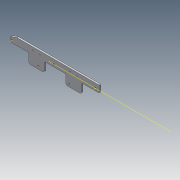
# Autodesk Inventor part: VP CAP SIDE COMP GUIDE
Saved by Autodesk Inventor 2020.3 (Build 243373000, 373)
## iProperties
RuleStatus: InUse
AfterDocSave0: file://Part Number Cleaner
Created: 2018-10-13
Material: DELRIN 100, WHITE (EXTRUDED)
Vendor: HHMI: JRC - ID&F
Document SubType Name: Modeling
Designer: arnoldj
Density: 1.42 g/cm^3
Appearance: Plastic (White)
DESIGN DEPARTMENT: HHMI: JRC - ID&F
ALTERED ITEM PART NUMBER: N/A
ALTERED ITEM VENDOR: N/A
ALTERED ITEM DESCRIPTION: N/A
Author: arnoldj
Revision Number: 0
Autodesk Inventor part; units mm, degrees
ref_plane "YZ Plane" through (0, 0, 0) normal (1, 0, 0) x (0, 1, 0)
ref_plane "XZ Plane" through (0, 0, 0) normal (0, 1, 0) x (-1, 0, 0)
sketch "Sketch1" plane through (0, 0, 0) normal (0, 0, 1) x (1, 0, 0)
  line L0 (0, 32.7219) -> (0, -62.9817) projected
  line L1 (-250.825, 0) -> (260.35, 0) projected
  line L2 (187.325, -9.525) -> (-177.8, -9.525)
  line L3 (-177.8, -9.525) -> (-177.8, 19.05)
  line L4 (-177.8, 19.05) -> (187.325, 19.05)
  line L5 (187.325, 19.05) -> (187.325, -9.525)
  line L6 (113.1316, -9.525) -> (49.6316, -9.525)
  line L7 (49.6316, -9.525) -> (49.6316, -49.3097)
  line L8 (49.6316, -49.3097) -> (113.1316, -49.3097)
  line L9 (113.1316, -49.3097) -> (113.1316, -9.525)
  line L10 (66.9925, 6.35) -> (95.5675, 6.35) construction
  line L11 (-171.45, -0.3175) -> (-171.45, 0.3175) construction
  line L12 (-173.99, -0.3175) -> (-173.99, 0.3175)
  line L13 (-168.91, 0.3175) -> (-168.91, -0.3175)
  arc A0 (-173.99, -0.3175) -> (-168.91, -0.3175) centre (-171.45, -0.3175) ccw
  arc A1 (-168.91, 0.3175) -> (-173.99, 0.3175) centre (-171.45, 0.3175) ccw
  line L14 (-63.5, -38.4175) -> (-63.5, -37.7825) construction
  line L15 (-66.04, -38.4175) -> (-66.04, -37.7825)
  line L16 (-60.96, -37.7825) -> (-60.96, -38.4175)
  arc A2 (-66.04, -38.4175) -> (-60.96, -38.4175) centre (-63.5, -38.4175) ccw
  arc A3 (-60.96, -37.7825) -> (-66.04, -37.7825) centre (-63.5, -37.7825) ccw
  line L17 (0, -0.3175) -> (0, 0.3175) construction
  line L18 (-2.54, -0.3175) -> (-2.54, 0.3175)
  line L19 (2.54, 0.3175) -> (2.54, -0.3175)
  arc A4 (-2.54, -0.3175) -> (2.54, -0.3175) centre (0, -0.3175) ccw
  arc A5 (2.54, 0.3175) -> (-2.54, 0.3175) centre (0, 0.3175) ccw
  line L20 (63.5, -38.4175) -> (63.5, -37.7825) construction
  line L21 (66.04, -38.4175) -> (66.04, -37.7825)
  line L22 (60.96, -37.7825) -> (60.96, -38.4175)
  arc A6 (60.96, -38.4175) -> (66.04, -38.4175) centre (63.5, -38.4175) ccw
  arc A7 (66.04, -37.7825) -> (60.96, -37.7825) centre (63.5, -37.7825) ccw
  line L23 (171.45, -0.3175) -> (171.45, 0.3175) construction
  line L24 (168.91, -0.3175) -> (168.91, 0.3175)
  line L25 (173.99, 0.3175) -> (173.99, -0.3175)
  arc A8 (168.91, -0.3175) -> (173.99, -0.3175) centre (171.45, -0.3175) ccw
  arc A9 (173.99, 0.3175) -> (168.91, 0.3175) centre (171.45, 0.3175) ccw
  point P0 (0, 0)
  point P1 (-171.45, 0)
  point P2 (0, 0)
  point P3 (63.5, 0)
  point P4 (171.45, 0)
  point P5 (81.28, 6.35)
  point P6 (63.5, -38.1)
  point P7 (-63.5, -38.1)
  dimension "d0" = 171.45
  dimension "d1" = 63.5
  dimension "d17" = 19.05
  dimension "d18" = 9.525
  dimension "d19" = 6.35
  dimension "d20" = 187.325
  dimension "d21" = 171.45
  dimension "d22" = 28.575
  dimension "d24" = 38.1
  dimension "d25" = 74.1934
  dimension "d26" = 63.5
  dimension "d42" = 81.28
  dimension "d48" = 63.5
  dimension "d49" = 6.35
  dimension "d50" = 2.54
  dimension "d51" = 0.635
  constraints: 58 end point, 20 point on circle, 20 tangent, 15 parallel, 10 centre point, 7 point on line, 6 midpoint, 4 equal radius, 3 horizontal, 3 perpendicular, 2 coincident, 1 horizontal alignment, 1 vertical, 1 vertical alignment
  measures "d0" distance from line of L0 point (-171.45, 0)
  measures "d1" distance from line of L0 point (63.5, 0)
  measures "d17" distance between parallel lines of L1 L4
  measures "d18" distance between parallel lines of L2 L1
  measures "d19" distance from line of point (-171.45, 0) L3
  measures "d20" distance between parallel lines of L5 L0
  measures "d21" distance from line of L0 point (171.45, 0)
  measures "d22" distance of L10.start L10.end
  measures "d24" distance of point (63.5, -38.1) point (63.5, 0)
  measures "d25" distance between parallel lines of L9 L5
  measures "d26" distance of L7.end L8.end
  measures "d42" distance from line of L0 point (81.28, 6.35)
  measures "d48" distance from line of L0 point (-63.5, -38.1)
  measures "d49" distance between parallel lines of L10 L1
  measures "d50" radius of A1
  measures "d51" distance of L12.start L12.end
extrude "Extrusion1" add sketch "Sketch1" against normal blind 6.35 contours L4 L5 L1 L25 A9 L24 L19 A5 L0 | L0 A5 L18 L1 L13 A1 L12 L3 L4 | A5 L19 L1 L0 | L0 L1 L18 A5 | L1 L19 A4 L0 | L0 A4 L18 L1 | L1 L12 A0 L13 L18 A4 L0 L2 L3 | L5 L2 L0 A4 L19 L1 L24 A8 L25 | L12 A1 L13 L1 | L1 L13 A0 L12 | L25 A8 L24 L1 | L1 L24 A9 L25
extrude "Extrusion2" add sketch "Sketch1" against normal up to surface (6.35 mm away) contours L9 L8 L7 L2 | A6 L22 A7 L21
hole "Hole3" at (66.9925, 6.35, 0) at (95.5675, 6.35, 0) direction (0, 0, -1) diameter 4.064 end through all
chamfer "Chamfer1" distance 25.4 angle 20 1 edges at (-177.8, 19.05, -3.175) measured on face at (-56.0917, 19.05, -2.1167)
fillet "Fillet1" radius 3.175 5 edges at (187.325, 19.05, -3.175) (187.325, -9.525, -3.175) (-177.8, -9.525, -3.175) (-177.8, 9.8052, -3.175) (-152.4, 19.05, -3.175)
fillet "Fillet2" radius 6.35 4 edges at (113.1316, -9.525, -3.175) (113.1316, -49.3097, -3.175) (49.6316, -49.3097, -3.175) (49.6316, -9.525, -3.175)
pattern_linear "Rectangular Pattern1" count 2 spacing 152.4 along (-1, 0, 0) of "Fillet2", "Hole3", "Extrusion2"
hole "Hole1" [suppressed]
extrude "Extrusion3" cut sketch "Sketch1" against normal up to next contours A5 L19 L1 L0 | L0 L1 L18 A5 | L1 L19 A4 L0 | L0 A4 L18 L1 | L12 A1 L13 L1 | L1 L13 A0 L12 | L25 A8 L24 L1 | L1 L24 A9 L25 | L15 A3 L16 A2 | A6 L22 A7 L21
body "Solid1"
